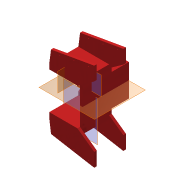
# Autodesk Inventor part: RearConnector
Saved by Autodesk Inventor 2016 (Build 200138000, 138)
## iProperties
Created: 2015-03-02
Part Number: RearConnector
Material: Generic
Document SubType Name: Modeling
Designer: Henke
Density: 1 g/cm^3
Appearance: Light Red
Author: Henke
Autodesk Inventor part; units mm, degrees
ref_plane "YZ Plane" through (0, 0, 0) normal (1, 0, 0) x (0, 1, 0)
ref_plane "XZ Plane" through (0, 0, 0) normal (0, 1, 0) x (-1, 0, 0)
ref_plane "XY Plane" through (0, 0, 0) normal (0, 0, 1) x (1, 0, 0)
sketch "Sketch1" plane through (0, 0, 0) normal (0, 0, 1) x (1, 0, 0)
  line L0 (0, 0) -> (35.7, 0)
  line L1 (35.7, 0) -> (35.7, 30.8)
  line L2 (35.7, 30.8) -> (0, 30.8)
  line L3 (0, 30.8) -> (0, 0)
  dimension "d0" = 35.7
  dimension "d1" = 30.8
  constraints: 8 end point, 2 parallel, 1 horizontal, 1 perpendicular
  measures "d0" distance of L1.end L2.end
  measures "d1" distance of L2.end L0.start
extrude "Extrusion1" add sketch "Sketch1" along normal blind 6
sketch "Sketch4" plane through (0, 0, 6) normal (0, 0, 1) x (1, 0, 0)
  line L0 (35.7, 30.8) -> (0, 30.8) projected
  line L1 (35.7, 0) -> (32.7, 0)
  line L2 (32.7, 0) -> (32.7, 30.8)
  line L3 (32.7, 30.8) -> (35.7, 30.8)
  line L4 (35.7, 30.8) -> (35.7, 0)
  point P0 (0, 0)
  dimension "d10" = 3
  constraints: 8 end point, 2 parallel, 1 horizontal, 1 perpendicular, 1 point on line
  measures "d10" distance between parallel lines of L4 L2
extrude "Extrusion3" add sketch "Sketch4" along normal blind 21.5
sketch "Sketch24" plane through (0, 30.8, 0) normal (0, 1, 0) x (1, 0, 0)
  line L0 (2, 15) -> (52.2252, 23.8561)
  line L1 (35.7, 0) -> (35.7, -27.5) projected
  line L2 (2, 15) -> (0, 0)
  line L3 (0, 0) -> (0, -6)
  line L4 (0, 0) -> (0, -6) projected
  line L5 (0, -6) -> (32.7, -6)
  line L6 (35.7, 0) -> (35.7, -27.5) projected
  line L7 (32.7, -6) -> (52.2252, 8)
  line L8 (52.2252, 23.8561) -> (52.2252, 8)
  line L9 (35.7, 0) -> (0, 0) projected
  circle A0 centre (45.2252, 19.9817) radius 0.5
  circle A1 centre (28.4835, 17.0296) radius 0.5
  circle A2 centre (11.7417, 14.0776) radius 0.5
  dimension "d152" = 51
  dimension "d153" = 80
  dimension "d155" = 15
  dimension "d159" = 17
  dimension "d160" = 1
  dimension "d161" = 1
  dimension "d162" = 2.6
  dimension "d163" = 2.6
  dimension "d164" = 7
  dimension "d165" = 2.6
  dimension "d166" = 17
  dimension "d167" = 2
  dimension "d168" = 8
  dimension "d169" = 1
  constraints: 12 end point, 3 centre point, 1 collinear, 1 parallel, 1 perpendicular
  measures "d152" distance of L0.start L0.end
  measures "d153" angle of L1 L0
  measures "d155" distance from line of L9 L0.start
  measures "d159" distance of A0.centre A1.centre
  measures "d160" diameter of A1
  measures "d161" diameter of A0
  measures "d162" distance from line of L0 A1.centre
  measures "d163" distance from line of L0 A0.centre
  measures "d164" distance from line of L8 A0.centre
  measures "d165" distance from line of L0 A2.centre
  measures "d166" distance of A1.centre A2.centre
  measures "d167" distance from line of L3 L0.start
  measures "d168" vertical distance of L1.start L7.end
  measures "d169" diameter of A2
extrude "Extrusion19" add sketch "Sketch24" along normal blind 3
ref_plane "Work Plane22" through (32.7, 15.4, 27.5) normal (0, 1, 0) x (1, 0, 0)
mirror "Mirror11" about plane through (32.7, 15.4, 27.5) normal (0, 1, 0) of "Extrusion19"
mirror "Mirror3" about plane through (34.2, 15.4, 27.5) normal (0, 0, 1) of "Extrusion1", "Extrusion3", "Extrusion19", "Mirror11"
sketch "Sketch28" plane through (35.7, 30.8, 51.1511) normal (0, 1, 0) x (1, 0, 0)
  circle A0 centre (-23.9583, -17.9266) radius 0.5 projected
  circle A1 centre (-7.2165, -20.8786) radius 0.5 projected
  circle A2 centre (9.5252, -23.8306) radius 0.5 projected
  circle A3 centre (-23.9583, 65.2287) radius 0.5 projected
  circle A4 centre (-7.2165, 68.1807) radius 0.5 projected
  circle A5 centre (9.5252, 71.1327) radius 0.5 projected
  line L0 (-35.7, 51.1511) -> (-33.7, 66.1511) projected
  line L1 (-33.7, 66.1511) -> (16.5252, 75.0071) projected
  line L2 (16.5252, 75.0071) -> (16.5252, 59.1511) projected
  line L3 (16.5252, 59.1511) -> (0, 47.3021) projected
  line L4 (0, 47.3021) -> (-3, 45.1511) projected
  line L5 (-3, 2.1511) -> (-3, 45.1511) projected
  line L6 (-3, 2.1511) -> (0, 0) projected
  line L7 (0, 47.3021) -> (0, 0) projected
  line L8 (-35.7, 51.1511) -> (0, 51.1511) projected
  line L9 (-35.7, 45.1511) -> (-35.7, 51.1511) projected
  line L10 (-3, 45.1511) -> (-35.7, 45.1511) projected
  line L11 (0, 51.1511) -> (0, 47.3021) projected
  line L12 (-35.7, 2.1511) -> (-3, 2.1511) projected
  line L13 (-35.7, -3.8489) -> (-35.7, 2.1511) projected
  line L14 (0, -3.8489) -> (-35.7, -3.8489) projected
  line L15 (0, 0) -> (0, -3.8489) projected
  line L16 (0, 0) -> (16.5252, -11.8489) projected
  line L17 (16.5252, -11.8489) -> (16.5252, -27.705) projected
  line L18 (16.5252, -27.705) -> (-33.7, -18.8489) projected
  line L19 (-33.7, -18.8489) -> (-35.7, -3.8489) projected
  line L20 (0, 47.3021) -> (0, 0) projected
  line L21 (0, 8.2511) -> (-3, 8.2511)
  line L22 (-3, 8.2511) -> (-3, 39.0511)
  line L23 (-3, 39.0511) -> (0, 39.0511)
  line L24 (0, 39.0511) -> (0, 8.2511)
  point P0 (-3, 23.6511)
  point P1 (-3, 23.6511)
  dimension "d205" = 30.8
  dimension "d206" = 3
  constraints: 8 end point, 2 midpoint, 2 parallel, 1 coincident, 1 horizontal, 1 perpendicular, 1 point on line
  measures "d205" distance of L21.end L22.end
  measures "d206" distance between parallel lines of L24 L22
extrude "Extrusion21" add sketch "Sketch28" along normal blind 23 contours L7 L21 L5 L23
sketch "Sketch29" plane through (32.7, 0, 6) normal (-1, 0, 0) x (0, 0, 1)
  line L0 (36.9, 30.8) -> (36.9, 53.8) projected
  line L1 (6.1, 33.8) -> (36.9, 33.8)
  line L2 (36.9, 33.8) -> (36.9, 36.8)
  line L3 (36.9, 36.8) -> (6.1, 36.8)
  line L4 (6.1, 36.8) -> (6.1, 33.8)
  line L5 (6.1, 53.8) -> (36.9, 53.8) projected
  line L6 (6.1, 30.8) -> (6.1, 53.8) projected
  point P0 (-6, 0)
  dimension "d207" = 3
  dimension "d208" = 17
  constraints: 8 end point, 2 parallel, 2 point on line, 1 horizontal, 1 perpendicular
  measures "d207" distance between parallel lines of L3 L1
  measures "d208" distance between parallel lines of L5 L3
extrude "Extrusion22" add sketch "Sketch29" along normal blind 36.1 contours L1 L4 L3 L0
sketch "Sketch30" plane through (-3.4, 0, 6) normal (-1, 0, 0) x (0, 0, 1)
  line L0 (6.1, 36.8) -> (36.9, 36.8) projected
  line L1 (36.9, 36.8) -> (36.9, 53.8) projected
  line L2 (6.1, 53.8) -> (36.9, 53.8) projected
  line L3 (6.1, 36.8) -> (6.1, 53.8) projected
  line L4 (6.1, 33.8) -> (36.9, 33.8) projected
  line L5 (36.9, 33.8) -> (36.9, 36.8) projected
  line L6 (36.9, 36.8) -> (6.1, 36.8) projected
  line L7 (6.1, 36.8) -> (6.1, 33.8) projected
  point P0 (-6, 0)
extrude "Extrusion23" add sketch "Sketch30" along normal blind 3
sketch "Sketch31" plane through (32.7, 30.8, 42.9) normal (0, 0, 1) x (1, 0, 0)
  line L0 (-39.1, 3) -> (3, 3)
  line L1 (3, 3) -> (3, 23)
  line L2 (3, 23) -> (-39.1, 23)
  line L3 (-39.1, 23) -> (-39.1, 3)
  circle A0 centre (-32.9, 15.3) radius 0.5
  circle A1 centre (-26.55, 8.875) radius 0.5
  circle A2 centre (-9.55, 8.875) radius 0.5
  circle A3 centre (-3.2, 15.3) radius 0.5
  line L4 (-32.9, 15.3) -> (-3.2, 15.3) construction
  line L5 (-26.55, 8.875) -> (-9.55, 8.875) construction
  line L6 (0, 6) -> (-36.1, 6) construction
  line L7 (-30.55, 23) -> (-5.55, 23)
  line L8 (-5.55, 23) -> (-5.55, 11.25)
  line L9 (-5.55, 11.25) -> (-30.55, 11.25)
  line L10 (-30.55, 11.25) -> (-30.55, 23)
  point P0 (-32.7, -30.8)
  point P1 (-18.05, 15.3)
  point P2 (-18.05, 23)
  point P3 (-18.05, 8.875)
  point P4 (-18.05, 11.25)
  dimension "d211" = 1
  dimension "d212" = 17
  dimension "d213" = 29.7
  dimension "d214" = 2.875
  dimension "d215" = 9.3
  dimension "d216" = 5.25
  dimension "d217" = 25
  constraints: 20 end point, 5 parallel, 4 centre point, 4 midpoint, 3 equal radius, 3 horizontal, 3 vertical alignment, 2 perpendicular, 1 point on line
  measures "d211" diameter of A0
  measures "d212" distance of L5.start L5.end
  measures "d213" distance of L4.start L4.end
  measures "d214" distance between parallel lines of L6 L5
  measures "d215" distance between parallel lines of L6 L4
  measures "d216" distance between parallel lines of L6 L9
  measures "d217" distance of L8.end L9.end
extrude "Extrusion24" add sketch "Sketch31" along normal blind 3 contours L3 L2 L10 L9 L8 L1 L0
ref_plane "Work Plane23" through (32.7, 0, 27.5) normal (0, 0, 1) x (1, 0, 0)
mirror "Mirror13" about plane through (32.7, 0, 27.5) normal (0, 0, 1) of "Extrusion24"
sketch "Sketch32" plane through (35.7, 30.8, 3.8489) normal (1, 0, 0) x (0, 0, -1)
  line L0 (3.8489, -30.8) -> (3.8489, 0) projected
  line L1 (3.8489, 0) -> (0, 0) projected
  line L2 (0, 0) -> (-8.2511, 0) projected
  line L3 (-8.2511, 0) -> (-8.2511, 3) projected
  line L4 (-8.2511, 3) -> (-5.2511, 3) projected
  line L5 (-5.2511, 3) -> (-5.2511, 23) projected
  line L6 (-5.2511, 23) -> (-42.0511, 23) projected
  line L7 (-42.0511, 3) -> (-42.0511, 23) projected
  line L8 (-39.0511, 3) -> (-42.0511, 3) projected
  line L9 (-39.0511, 0) -> (-39.0511, 3) projected
  line L10 (-39.0511, 0) -> (-47.3021, 0) projected
  line L11 (-51.1511, 0) -> (-47.3021, 0) projected
  line L12 (-51.1511, -30.8) -> (-51.1511, 0) projected
  line L13 (-47.3021, -30.8) -> (-51.1511, -30.8) projected
  line L14 (0, -30.8) -> (-47.3021, -30.8) projected
  line L15 (3.8489, -30.8) -> (0, -30.8) projected
  line L16 (-39.0511, 0) -> (-45.1511, 0)
  line L17 (-45.1511, 0) -> (-45.1511, 3)
  line L18 (-45.1511, 3) -> (-39.0511, 3)
  line L19 (-39.0511, 3) -> (-39.0511, 0)
  line L20 (-8.2511, 0) -> (-2.1511, 0)
  line L21 (-2.1511, 0) -> (-2.1511, 3)
  line L22 (-2.1511, 3) -> (-8.2511, 3)
  line L23 (-8.2511, 3) -> (-8.2511, 0)
  constraints: 16 end point, 4 parallel, 2 horizontal, 2 perpendicular
extrude "Extrusion25" add sketch "Sketch32" against normal up to surface (35.7 mm away) contours L2 L3 L4 L22 L21 | L17 L18 L8 L9 L10
chamfer "Chamfer9" distance 2 angle 45 2 edges at (16.35, 30.8, 12.1) (16.35, 30.8, 42.9)
sketch "Sketch33" plane through (32.7, 30.8, 49) normal (0, 1, 0) x (1, 0, 0)
  line L0 (3, 0) -> (3, -2.1511) projected
  line L1 (3, 0) -> (0, 0) projected
  line L2 (3, -2.1511) -> (0, 0) projected
  line L3 (3, 45.1511) -> (0, 43) projected
  line L4 (3, 45.1511) -> (3, 43) projected
  line L5 (0, 43) -> (3, 43) projected
  point P0 (-32.7, 49)
extrude "Extrusion26" add sketch "Sketch33" along normal up to surface (3 mm away)
chamfer "Chamfer10" distance 2 angle 45 5 edges at (-6.4, 33.8, 27.5) (-3.2, 33.8, 45.9) (-6.4, 43.8, 45.9) (-3.2, 33.8, 9.1) (-6.4, 43.8, 9.1)
ref_plane "Work Plane3" through (17.85, 0, 49) normal (-1, 0, 0) x (0, 1, 0)
ref_plane "Work Plane4" through (35.7, 10.55, 49) normal (0, -1, 0) x (-1, 0, 0)
body "Solid1"
